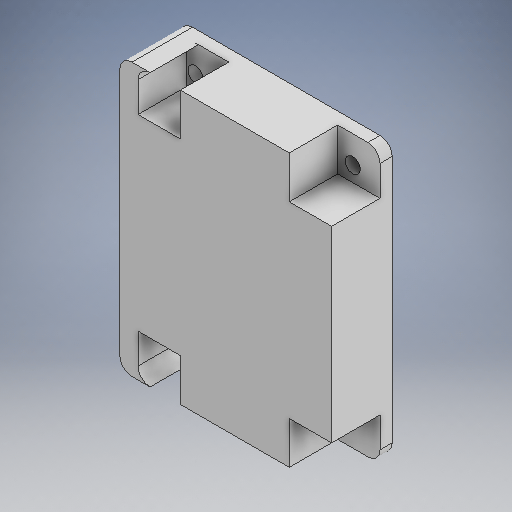
# Autodesk Inventor part: Sensor Housing
Saved by Autodesk Inventor 2025.3 (Build 293356000, 356)
## iProperties
Created: 2026-04-06
Part Number: Sensor Housing
Material: Generic
Document SubType Name: Modeling
Designer: user
Density: 1 g/cm^3
Appearance: Default
Author: user
Autodesk Inventor part; units mm, degrees
ref_plane "YZ Plane" through (0, 0, 0) normal (1, 0, 0) x (0, 1, 0)
ref_plane "XZ Plane" through (0, 0, 0) normal (0, 1, 0) x (-1, 0, 0)
ref_plane "XY Plane" through (0, 0, 0) normal (0, 0, 1) x (1, 0, 0)
sketch "Sketch1" plane through (0, 0, 0) normal (0, 0, 1) x (1, 0, 0)
  line L0 (0, 0) -> (35, 0)
  line L1 (35, 0) -> (35, 45)
  line L2 (0, 45) -> (35, 45) construction
  circle A0 centre (4.5, 40.5) radius 1.25
  line L3 (17.5, 50) -> (17.5, 0) construction
  circle A1 centre (30.5, 40.5) radius 1.25
  line L4 (0, 45) -> (0, 0)
  line L5 (0, 22.5) -> (35, 22.5) construction
  circle A2 centre (4.5, 4.5) radius 1.25
  circle A3 centre (30.5, 4.5) radius 1.25
  line L6 (8.5, 3.5) -> (26.5, 3.5)
  line L7 (26.5, 3.5) -> (26.5, 43.5)
  line L8 (26.5, 43.5) -> (8.5, 43.5)
  line L9 (8.5, 43.5) -> (8.5, 3.5)
  line L10 (8.5, 3.5) -> (10, 3.5)
  line L11 (8.5, 4.5) -> (8.5, 3.5)
  line L12 (9.5, 4.5) -> (9.5, 43.5)
  line L13 (8.5, 4.5) -> (11, 4.5)
  line L14 (11, 4.5) -> (11, 3.5)
  line L15 (25.5, 4.5) -> (25.5, 43.5)
  line L16 (26.5, 4.5) -> (24, 4.5)
  line L17 (24, 4.5) -> (24, 3.5)
  line L18 (0, 45) -> (35, 45)
  line L19 (0, 45) -> (0, 0)
  point P0 (11, 4)
  point P1 (24, 4)
  point P2 (9.5, 4.5)
  point P3 (25.5, 4.5)
  point P4 (24, 3.5)
  dimension "d5" = 2.5
  dimension "d6" = 4.5
  dimension "d8" = 2.5
  dimension "d9" = 18
  dimension "d10" = 40
  dimension "d11" = 3.5
  dimension "d19" = 1
  dimension "d26" = 8
  dimension "d27" = 2.5
  dimension "d28" = 35
  dimension "d29" = 1.5
  dimension "d30" = 26
  dimension "d31" = 9
  dimension "d54" = 45
  constraints: 40 end point, 8 symmetric about line, 5 horizontal, 5 midpoint, 4 centre point, 4 perpendicular, 3 parallel, 2 point on line, 2 vertical, 1 coincident, 2 other
  measures "d5" diameter of A0
  measures "d6" distance from line of L2 A0.centre
  measures "d8" diameter of A3
  measures "d9" distance of L8.end L7.end
  measures "d10" distance of L7.end L6.end
  measures "d11" distance between parallel lines of L0 L6
  measures "d19" distance of L16.end L17.end
  measures "d26" distance between parallel lines of L3 L12
  measures "d27" distance of L11.start L13.end
  measures "d28" distance of L2.start L1.end
  measures "d29" distance between parallel lines of L8 L2
  measures "d30" distance of A1.centre A0.centre
  measures "d31" distance between parallel lines of L3 L7
  measures "d54" distance of L2.start L0.start
extrude "Extrusion1" add sketch "Sketch1" along normal blind 2 contours L4 L18 L1 L0 | L9 L13 L14 L6 | L9 L8 L12 L13 | L14 L13 L12 L8 L15 L16 L17 L6 | L17 L16 L7 L6 | L8 L7 L16 L15
extrude "Extrusion2" add sketch "Sketch1" against normal blind 8 contours L9 L13 L14 L6 | L9 L8 L12 L13 | L17 L16 L7 L6 | L8 L7 L16 L15
fillet "Fillet1" radius 2 2 edges at (26.5, 3.5, -4) (8.5, 3.5, -4)
fillet "Fillet2" radius 2 2 edges at (25.5, 43.5, -4) (9.5, 43.5, -4)
fillet "Fillet3" radius 2 4 edges at (35, 45, 1) (0, 45, 1) (0, 0, 1) (35, 0, 1)
thicken "Thicken1" operation add thickness 8 both sides no extend neighbours no toward (0, 0, -1) faces at (19.6667, 29.3453, 0)
sketch "Sketch3" plane through (33, 0, -8) normal (0, 0, -1) x (-1, 0, 0)
  line L0 (15, 49) -> (15, -1) construction
  line L1 (-2.5, 20) -> (32.5, 20) construction
  line L2 (6, 2.5) -> (24, 2.5)
  line L3 (24, 2.5) -> (24, 42.5)
  line L4 (24, 42.5) -> (6, 42.5)
  line L5 (6, 42.5) -> (6, 2.5)
  line L6 (6, 2.5) -> (7.5, 2.5)
  line L7 (6, 3.5) -> (6, 2.5)
  line L8 (7, 3.5) -> (7, 42.5)
  line L9 (6, 3.5) -> (8.5, 3.5)
  line L10 (8.5, 3.5) -> (8.5, 2.5)
  line L11 (23, 3.5) -> (23, 42.5)
  line L12 (24, 3.5) -> (21.5, 3.5)
  line L13 (21.5, 3.5) -> (21.5, 2.5)
  line L14 (31, 0) -> (0, 0) projected
  point P0 (33, 0)
  point P1 (8.5, 3)
  point P2 (21.5, 3)
  point P3 (7, 3.5)
  dimension "d36" = 18
  dimension "d37" = 40
  dimension "d38" = 1
  dimension "d39" = 8
  dimension "d40" = 2.5
  dimension "d41" = 9
  dimension "d42" = 2.5
  dimension "d43" = 7
  dimension "d44" = 8.5
  constraints: 28 end point, 5 symmetric about line, 3 horizontal, 2 midpoint, 2 parallel, 2 point on line, 1 perpendicular, 1 vertical
  measures "d36" distance of L5.start L3.end
  measures "d37" distance of L3.end L3.start
  measures "d38" distance of L12.end L13.end
  measures "d39" distance between parallel lines of L0 L8
  measures "d40" distance of L9.start L10.start
  measures "d41" distance between parallel lines of L0 L3
  measures "d42" distance between parallel lines of L14 L2
  measures "d43" distance from line of L14.end L8
  measures "d44" horizontal distance of L14.end point (8.5, 3)
extrude "Extrusion3" cut sketch "Sketch3" against normal blind 8 contours L10 L9 L8 L4 L11 L12 L13 L2
sketch "Sketch4" plane through (0, 0, 2) normal (0, 0, 1) x (1, 0, 0)
  line L0 (10, 42.5) -> (10, 3.5) projected
  line L1 (5, 45) -> (10, 45)
  line L2 (10, 45) -> (10, 38)
  line L3 (10, 38) -> (3, 38)
  line L4 (3, 38) -> (3, 43)
  line L5 (33, 45) -> (28, 45)
  line L6 (28, 45) -> (28, 38)
  line L7 (28, 38) -> (35, 38)
  line L8 (35, 38) -> (35, 43)
  arc A0 (5, 45) -> (3, 43) centre (5, 43) ccw
  arc A1 (35, 43) -> (33, 45) centre (33, 43) ccw
  line L9 (0, 0) -> (0, 45)
  line L10 (35, 2) -> (35, 43) projected
  line L11 (35, 22.5) -> (39, 22.5)
  line L12 (10, 2.5) -> (10, 41.5)
  line L13 (5, 0) -> (10, 0)
  line L14 (10, 0) -> (10, 7)
  line L15 (10, 7) -> (3, 7)
  line L16 (3, 7) -> (3, 2)
  line L17 (33, 0) -> (28, 0)
  line L18 (28, 0) -> (28, 7)
  line L19 (28, 7) -> (35, 7)
  line L20 (35, 7) -> (35, 2)
  arc A2 (3, 2) -> (5, 0) centre (5, 2) ccw
  arc A3 (33, 0) -> (35, 2) centre (33, 2) ccw
  line L21 (0, 45) -> (0, 0)
  line L22 (35, 43) -> (35, 2)
  point P0 (35, 45)
  point P1 (35, 0)
  point P2 (35, 7)
  point P3 (0, 10)
  point P4 (0, 2)
  dimension "d47" = 7
  dimension "d48" = 2
  dimension "d49" = 2
  constraints: 42 end point, 18 symmetric about line, 10 point on line, 8 point on circle, 4 centre point, 4 parallel, 4 perpendicular, 4 tangent, 3 horizontal, 1 midpoint, 1 vertical, 2 other
  measures "d47" distance of L5.end L6.end
  measures "d48" radius of A0
  measures "d49" radius of A1
extrude "Extrusion4" cut sketch "Sketch4" against normal blind 8
sketch "Sketch6" plane through (11.5, 2.5, -8) normal (0, 1, 0) x (1, 0, 0)
  line L0 (23.5, -10) -> (16.5, -10) projected
  line L1 (14.5, 0) -> (-1.5, 0) projected
  line L2 (16.5, -10) -> (-1.5, -10)
  line L3 (-1.5, -10) -> (-1.5, 0)
  line L4 (-1.5, 0) -> (16.5, 0)
  line L5 (16.5, 0) -> (16.5, -10)
  point P0 (-11.5, -8)
  point P1 (13.5, 0)
  constraints: 8 end point, 2 parallel, 1 horizontal, 1 perpendicular
extrude "Extrusion5" [suppressed]
body "Solid1"
